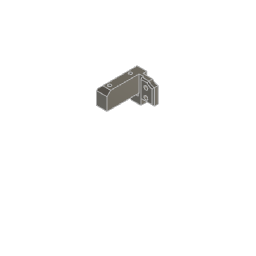
BLTouchBracket (Autodesk Fusion 360 design; units mm, degrees)
Autodesk Fusion 360 part; units mm, degrees
note: some values were not read from the file. Set by a fixed rule: which sketch regions a step uses.
sketch "Sketch1" plane through (0, 0, 0) normal (0, -1, 0) x (1, 0, 0)
  circle A0 centre (6, 20) radius 1.5
  circle A1 centre (6, 27) radius 1.5
  arc A2 (61, 37) -> (51, 47) centre (51, 37) ccw
  line L0 (51, 47) -> (10, 47)
  arc A3 (10, 47) -> (0, 37) centre (10, 37) ccw
  line L1 (0, 37) -> (0, 0)
  line L2 (0, 0) -> (61, 0)
  line L3 (61, 0) -> (61, 37)
  line L4 (-10, 16.6) -> (12, 16.6)
  line L5 (12, 16.6) -> (12, 32)
  line L6 (12, 32) -> (-10, 32)
  line L7 (-10, 32) -> (-10, 16.6)
  circle A4 centre (12, 35) radius 5
  circle A5 centre (12, 35) radius 5.4
  line L8 (0, 18.6) -> (-10, 18.6)
  line L9 (0, 18.6) -> (1.9728, 16.6)
  dimension "d1" = 0.4
  dimension "d4" = 12
  dimension "d5" = 10
  dimension "d6" = 15
  dimension "d7" = 15.4
  dimension "d45" = 2
  constraint horizontal L4
  constraint vertical L5
  constraint horizontal L6
  constraint vertical L7
  constraint coincident L7 L8.end
  constraint perpendicular L7 L8
  constraint coincident L4 L9.end
  measures "d4" distance of L1 L5
  measures "d5" distance of L1 L7
  measures "d6" distance of L0 L6
  measures "d7" distance of L4.start L6.end
  measures "d45" distance of L4 L8
extrude "Extrude1" add sketch "Sketch1" along normal blind 2 contours L1 L4 L9 | L1 L4 L5 L6 A5 L9 | L1 L6 L7 L8
sketch "Sketch7" plane through (0, -2, 0) normal (0, -1, 0) x (1, 0, 0)
  circle A0 centre (6, 20) radius 1.5
  circle A1 centre (6, 27) radius 1.5
  line L0 (7.51, 32) -> (-10, 32)
  line L1 (-10, 32) -> (-10, 18.6)
  line L2 (0, 16.6) -> (12, 16.6)
  line L3 (12, 16.6) -> (12, 29.6)
  arc A2 (7.51, 32) -> (12, 29.6) centre (12, 35) ccw
  circle A3 centre (12, 35) radius 5
  circle A4 centre (6, 20) radius 1.5
  circle A5 centre (6, 27) radius 1.5
  arc A6 (61, 37) -> (51, 47) centre (51, 37) ccw
  line L4 (51, 47) -> (10, 47)
  arc A7 (10, 47) -> (0, 37) centre (10, 37) ccw
  line L5 (0, 37) -> (0, 0)
  line L6 (0, 0) -> (61, 0)
  line L7 (61, 0) -> (61, 37)
  line L8 (0, 32) -> (0, 16.6)
  line L9 (0, 32) -> (2, 32)
  line L10 (2, 32) -> (2, 16.6)
  line L11 (2, 16.6) -> (0, 16.6)
  line L12 (0, 16.6) -> (0, 32)
  line L13 (2, 32) -> (12, 32)
  line L14 (12, 32) -> (12, 16.6)
  line L15 (12, 16.6) -> (2, 16.6)
  line L16 (2, 16.6) -> (2, 32)
  line L17 (-10, 18.6) -> (0, 18.6)
  line L18 (0, 18.6) -> (0, 16.6)
  dimension "d39" = 2
  constraint coincident L0 L8.start
  constraint coincident L5 L8.start
  constraint coincident L2 L8.end
  constraint coincident L5 L2.start
  constraint horizontal L9
  constraint vertical L10
  constraint horizontal L11
  constraint vertical L12
  constraint horizontal L13
  constraint vertical L14
  constraint horizontal L15
  constraint vertical L16
  constraint coincident L2.end L3.start
  measures "d39" distance of L8.start L9.end
extrude "Extrude6" add sketch "Sketch7" along normal blind 2 contours L0 L2 L3 A2 L10 L13 L14 L15 L16
sketch "Sketch3" plane through (0, -2, 0) normal (0, -1, 0) x (1, 0, 0)
  line L0 (2, 32) -> (-10, 32)
  line L1 (-10, 32) -> (-10, 18.6)
  line L2 (0, 16.6) -> (2, 16.6)
  line L3 (-10, 32) -> (-1.5423, 32)
  line L4 (-1.5423, 32) -> (-1.5423, 18.6)
  line L5 (-1.5423, 18.6) -> (-10, 18.6)
  line L6 (-10, 18.6) -> (-10, 32)
  line L7 (2, 16.6) -> (2, 32)
  line L8 (-10, 18.6) -> (0, 18.6)
  line L9 (0, 18.6) -> (0, 16.6)
  constraint horizontal L3
  constraint vertical L4
  constraint horizontal L5
  constraint vertical L6
  constraint coincident L0.end L1.start
extrude "Extrude2" add sketch "Sketch3" along normal blind 26 contours L0 L1 L3 L4 L5 L6 L8
sketch "Sketch5" plane through (0, 0, 0) normal (0, 1, 0) x (-1, 0, 0)
  circle A0 centre (-6, 27) radius 1.5
  circle A1 centre (-6, 20) radius 1.5
  line L0 (10, 32) -> (-7.51, 32)
  arc A2 (-12, 29.6) -> (-7.51, 32) centre (-12, 35) ccw
  line L1 (-12, 29.6) -> (-12, 16.6)
  line L2 (-12, 16.6) -> (0, 16.6)
  line L3 (10, 18.6) -> (10, 32)
  circle A3 centre (-6, 20) radius 1.5
  circle A4 centre (-6, 27) radius 1.5
  arc A5 (-51, 47) -> (-61, 37) centre (-51, 37) ccw
  line L4 (-61, 37) -> (-61, 0)
  line L5 (-61, 0) -> (0, 0)
  line L6 (0, 0) -> (0, 37)
  arc A6 (0, 37) -> (-10, 47) centre (-10, 37) ccw
  line L7 (-10, 47) -> (-51, 47)
  line L8 (10, 32) -> (0.2, 32)
  line L9 (0.2, 32) -> (0.2, 16.6)
  line L10 (0.2, 16.6) -> (10, 16.6)
  line L11 (10, 16.6) -> (10, 32)
  line L12 (0, 16.6) -> (0, 18.6)
  circle A7 centre (-6, 20) radius 1.5
  circle A8 centre (-6, 27) radius 1.5
  line L13 (10, 32) -> (-7.51, 32)
  arc A9 (-12, 29.6) -> (-7.51, 32) centre (-12, 35) ccw
  line L14 (-12, 29.6) -> (-12, 16.6)
  line L15 (-12, 16.6) -> (0, 16.6)
  line L16 (0, 16.6) -> (0, 18.6)
  line L17 (0, 18.6) -> (10, 18.6)
  line L18 (10, 18.6) -> (10, 32)
  line L19 (0, 18.6) -> (10, 18.6)
  dimension "d26" = 0.2
  constraint horizontal L8
  constraint vertical L9
  constraint horizontal L10
  constraint vertical L11
  constraint coincident L2 L9.end
  constraint coincident L0.start L3.end
  measures "d26" distance of L6 L9
extrude "Extrude4" add sketch "Sketch5" along normal blind 3 contours L0 L3 L8 L9 L11 L13 L17 L18 L19
sketch "Sketch4" plane through (0, 0, 18.6) normal (0, 0, -1) x (1, 0, 0)
  line L0 (0, 2) -> (-1.5423, 2)
  line L1 (-1.5423, 2) -> (-1.5423, 28)
  line L2 (-1.5423, 28) -> (-10, 28)
  line L3 (-10, 28) -> (-10, -3)
  ellipse E0 centre (-5.5, 13.5) end of major axis (-5.5, 26.55) minor radius 3.0346
  line L4 (-5.5, 0.45) -> (-5.5, 26.55)
  line L5 (-2.4654, 13.5) -> (-8.5346, 13.5)
  circle A0 centre (-5.5, 22) radius 1.25
  circle A1 centre (-5.5, 5) radius 1.25
  line L6 (-10, -3) -> (-0.2, -3)
  line L7 (-0.2, -3) -> (-0.2, 0)
  line L8 (-0.2, 0) -> (0, 0)
  line L9 (0, 0) -> (0, 2)
  dimension "d18" = 26.1
  dimension "d19" = 2.5
  dimension "d21" = 8.5
  dimension "d24" = 8.5
  dimension "d35" = 4.5
  dimension "d47" = 6
  constraint vertical L4
  constraint coincident E0 L4.start
  constraint coincident E0 L4.end
  constraint coincident E0 L5.start
  constraint coincident E0 L5.end
  constraint coincident L4 A0.centre
  constraint coincident L4 A1.centre
  constraint equal A0 A1
  measures "d18" distance of E0
  measures "d19" diameter of A0
  measures "d21" distance of L5 A0.centre
  measures "d24" distance of E0.centre A1.centre
  measures "d35" distance of L3 L4
  measures "d47" distance of L2 A0.centre
extrude "Extrude3" cut sketch "Sketch4" against normal blind 18 contours L4 A0 | L4 A0 | L4 A1 | L4 A1
sketch "Sketch6" plane through (-10, 0, 0) normal (-1, 0, 0) x (0, -1, 0)
  line L0 (-3, 18.6) -> (28, 18.6)
  line L1 (28, 18.6) -> (28, 32)
  line L2 (28, 32) -> (-3, 32)
  line L3 (-3, 32) -> (-3, 18.6)
  line L4 (2.4, 25.8) -> (7.6, 25.8)
  line L5 (7.6, 25.8) -> (7.6, 23.4)
  line L6 (7.6, 23.4) -> (2.4, 23.4)
  line L7 (2.4, 23.4) -> (2.4, 25.8)
  line L8 (19.4, 25.8) -> (24.6, 25.8)
  line L9 (24.6, 25.8) -> (24.6, 23.4)
  line L10 (24.6, 23.4) -> (19.4, 23.4)
  line L11 (19.4, 23.4) -> (19.4, 25.8)
  line L12 (7.6, 24.6) -> (19.4, 24.6) construction
  point P0 (5, 23.4)
  point P1 (22, 23.4)
  dimension "d29" = 5.2
  dimension "d30" = 2.4
  dimension "d49" = 6
  dimension "d60" = 6
  constraint horizontal L4
  constraint vertical L5
  constraint horizontal L6
  constraint vertical L7
  constraint horizontal L8
  constraint vertical L9
  constraint horizontal L10
  constraint vertical L11
  constraint equal L4 L8
  constraint equal L5 L9
  constraint midpoint L5 L12.start
  constraint midpoint L11 L12.end
  constraint horizontal L12
  constraint midpoint L6 P0
  constraint midpoint L10 P1
  measures "d29" distance of L4.start L4.end
  measures "d30" distance of L4.start L6.end
  measures "d49" distance of L0 L12
  measures "d60" distance of L1 P1
extrude "Extrude5" cut sketch "Sketch6" against normal blind 7 contours L4 L5 L6 L7 | L8 L9 L10 L11
box "BoxPrimitive1" add length 5 width 10 height 8 placed x (0, -1, 0) y (-1, 0, 0) z (0, 0, -1) at (0, 3, 18.6)
sketch "Sketch9" plane through (0, -2, 0) normal (0, -1, 0) x (1, 0, 0)
  line L0 (-1.5423, 32) -> (-1.5423, 18.6)
  line L1 (-1.5423, 18.6) -> (-10, 18.6)
  line L2 (-10, 18.6) -> (-10, 10.6)
  line L3 (-10, 10.6) -> (0, 10.6)
  line L4 (0, 10.6) -> (0, 16.6)
  line L5 (0, 16.6) -> (2, 16.6)
  line L6 (2, 16.6) -> (2, 32)
  line L7 (2, 32) -> (-1.5423, 32)
  line L8 (-9.0424, 18.6) -> (-2.2185, 18.6)
  line L9 (-2.2185, 18.6) -> (-2.2185, 16.1)
  line L10 (-2.2185, 16.1) -> (-9.0424, 16.1)
  line L11 (-9.0424, 16.1) -> (-9.0424, 18.6)
  line L12 (-10, 18.6) -> (-1.5423, 18.6)
  line L13 (-1.5423, 18.6) -> (-1.5423, 32)
  line L14 (-1.5423, 32) -> (-10, 32)
  line L15 (-10, 32) -> (-10, 18.6)
  point P0 (-5.7711, 18.6)
  point P1 (-5.5, 18.6)
  dimension "d57" = 2.5
  constraint horizontal L8
  constraint vertical L9
  constraint horizontal L10
  constraint vertical L11
  constraint coincident L1 L8.start
  constraint midpoint L12 P0
  measures "d57" distance of L8.start L10.end
extrude "Extrude7" cut sketch "Sketch9" against normal blind 3 contours L1 L8 L9 L10 L11 L12
chamfer "Chamfer3" distance 1 angle 45 4 edges at (4.755, -4, 32) (9.4544, -4, 30.2376) (12, -4, 23.1) (7, -4, 16.6)
chamfer "Chamfer3" distance 2 angle 45 1 edges at (-10, 0.5, 10.6)
chamfer "Chamfer3" distance 3 angle 45 1 edges at (-5.7711, -28, 32)
chamfer "Chamfer3" distance 2 angle 45 1 edges at (-10, -12.5, 32)
equation "d21 = ( 17 / 2 ) * 1 mm"
equation "d24 = d21"
